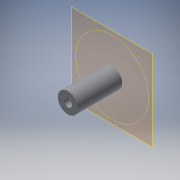
# Autodesk Inventor part: Inner Gear Extruded
Saved by Autodesk Inventor 2016 (Build 200138000, 138)
## iProperties
Created: 2016-04-25
Part Number: Inner Gear Extruded
Material: Generic
Document SubType Name: Modeling
Designer: rubenjm
Density: 1 g/cm^3
Appearance: Default
Author: rubenjm
Autodesk Inventor part; units mm, degrees
ref_plane "YZ Plane" through (0, 0, 0) normal (1, 0, 0) x (0, 1, 0)
ref_plane "XZ Plane" through (0, 0, 0) normal (0, 1, 0) x (-1, 0, 0)
ref_plane "XY Plane" through (0, 0, 0) normal (0, 0, 1) x (1, 0, 0)
sketch "Sketch1" plane through (0, 0, 0) normal (0, 0, 1) x (1, 0, 0)
  circle A0 centre (0, 0) radius 17.4793 construction
  circle A1 centre (0, 0) radius 23.2285 construction
  circle A2 centre (0, 0) radius 6.35
  circle A3 centre (0, 0) radius 2.5019
  dimension "d0" = 46.4569
  dimension "d1" = 34.9586
  dimension "d2" = 12.7
  dimension "d3" = 5.0038
  constraints: 4 centre point, 4 coincident
  measures "d0" diameter of A1
  measures "d1" diameter of A0
  measures "d2" diameter of A2
  measures "d3" diameter of A3
extrude "Extrusion1" add sketch "Sketch1" along normal blind 27.8384
sketch "Sketch2" plane through (0, 0, 0) normal (1, 0, 0) x (0, 1, 0)
  line L0 (0, 0) -> (0, 27.8384) construction
  line L1 (6.35, 27.8384) -> (-6.35, 27.8384) construction
  circle A0 centre (0, 13.9192) radius 2.65
  dimension "d6" = 5.3
  constraints: 2 end point, 2 midpoint, 1 centre point
  measures "d6" diameter of A0
extrude "Extrusion2" cut sketch "Sketch2" against normal through all
ref_plane "Work Plane1" through (0, 0, 0) normal (0, 0, 1) x (1, 0, 0)
sketch "Sketch3" plane through (0, 0, 0) normal (0, 0, 1) x (1, 0, 0)
  circle A0 centre (0, 0) radius 22.9615 construction
  constraints: 1 centre point, 1 coincident
body "Solid1"
